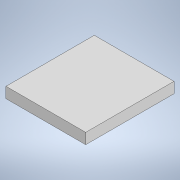
# Autodesk Inventor part: FishTankLid
Saved by Autodesk Inventor 2020 (Build 240168000, 168)
## iProperties
Created: 2020-03-05
Part Number: FishTankLid
Material: Generic
Document SubType Name: Modeling
Designer: jared.jones280
Density: 1 g/cm^3
Appearance: Default
Author: jared.jones280
Autodesk Inventor part; units mm, degrees
ref_plane "YZ Plane" through (0, 0, 0) normal (1, 0, 0) x (0, 1, 0)
ref_plane "XZ Plane" through (0, 0, 0) normal (0, 1, 0) x (-1, 0, 0)
ref_plane "XY Plane" through (0, 0, 0) normal (0, 0, 1) x (1, 0, 0)
sketch "Sketch1" plane through (0, 0, 0) normal (0, 1, 0) x (-1, 0, 0)
  line L0 (0, 0) -> (-205.994, 0)
  line L1 (-205.994, 0) -> (-205.994, -228.854)
  line L2 (-205.994, -228.854) -> (0, -228.854)
  line L3 (0, -228.854) -> (0, 0)
  line L4 (-209.169, -232.029) -> (3.175, -232.029)
  line L5 (3.175, -232.029) -> (3.175, 3.175)
  line L6 (3.175, 3.175) -> (-209.169, 3.175)
  line L7 (-209.169, 3.175) -> (-209.169, -232.029)
  dimension "d0" = 205.994
  dimension "d1" = 228.854
  dimension "d2" = 3.175
  dimension "d3" = 3.175
  dimension "d4" = 3.175
  dimension "d5" = 3.175
  constraints: 16 end point, 4 parallel, 2 horizontal, 2 perpendicular, 1 coincident
  measures "d0" distance of L2.end L1.end
  measures "d1" distance of L1.end L0.end
  measures "d2" horizontal distance of L5.end point (0, 0)
  measures "d3" horizontal distance of point (0, 0) L5.end
  measures "d4" horizontal distance of L1.end L4.start
  measures "d5" horizontal distance of L1.end L4.start
extrude "Extrusion2" add sketch "Sketch1" along normal blind 25.4
sketch "Sketch2" plane through (0, 25.4, 0) normal (0, 1, 0) x (1, 0, 0)
  line L0 (-3.175, 232.029) -> (-3.175, -3.175) projected
  line L1 (-3.175, -3.175) -> (209.169, -3.175) projected
  line L2 (209.169, -3.175) -> (209.169, 232.029) projected
  line L3 (209.169, 232.029) -> (-3.175, 232.029) projected
  point P0 (0, 0)
extrude "Extrusion3" add sketch "Sketch2" along normal blind 3.175
sketch "Sketch4" plane through (0, 25.4, 0) normal (0, -1, 0) x (1, 0, 0)
  point P0 (0, 0)
body "Solid2"
